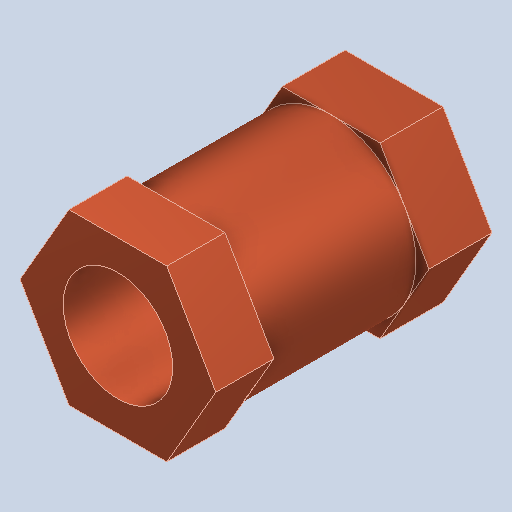
# Autodesk Inventor part: AcopleIntermedio
Saved by Autodesk Inventor 2023 (Build 270158000, 158)
## iProperties
Created: 2022-11-04
Part Number: AcopleIntermedio
Material: Copper
Document SubType Name: Modeling
Designer: Daniel Peña
Density: 8.94 g/cm^3
Appearance: Copper - Satin
Author: Daniel Peña
Autodesk Inventor part; units mm, degrees
ref_plane "YZ Plane" through (0, 0, 0) normal (1, 0, 0) x (0, 1, 0)
ref_plane "XZ Plane" through (0, 0, 0) normal (0, 1, 0) x (-1, 0, 0)
ref_plane "XY Plane" through (0, 0, 0) normal (0, 0, 1) x (1, 0, 0)
sketch "Sketch1" plane through (0, 0, 0) normal (0, 0, 1) x (1, 0, 0)
  line L0 (10.1036, 0) -> (5.0518, -8.75)
  line L1 (5.0518, -8.75) -> (-5.0518, -8.75)
  line L2 (-5.0518, -8.75) -> (-10.1036, 0)
  line L3 (-10.1036, 0) -> (-5.0518, 8.75)
  line L4 (-5.0518, 8.75) -> (5.0518, 8.75)
  line L5 (5.0518, 8.75) -> (10.1036, 0)
  circle A0 centre (0, 0) radius 5.5
  dimension "d0" = 17.5
  dimension "d1" = 11
  constraints: 12 end point, 2 coincident, 1 centre point, 13 other
  measures "d0" distance between parallel lines of L1 L4
  measures "d1" diameter of A0
extrude "Extrusion1" add sketch "Sketch1" along normal blind 6.5
sketch "Sketch2" plane through (0, 0, 6.5) normal (0, 0, 1) x (1, 0, 0)
  circle A0 centre (0, 0) radius 8.75
  circle A1 centre (0, 0) radius 5.65
  dimension "d4" = 17.5
  dimension "d5" = 11.3
  constraints: 2 centre point, 2 coincident
  measures "d4" diameter of A0
  measures "d5" diameter of A1
extrude "Extrusion2" add sketch "Sketch2" along normal blind 16
sketch "Sketch3" plane through (0, 0, 22.5) normal (0, 0, 1) x (1, 0, 0)
  circle A0 centre (0, 0) radius 5.65 projected
  line L0 (10.1036, 0) -> (5.0518, -8.75)
  line L1 (5.0518, -8.75) -> (-5.0518, -8.75)
  line L2 (-5.0518, -8.75) -> (-10.1036, 0)
  line L3 (-10.1036, 0) -> (-5.0518, 8.75)
  line L4 (-5.0518, 8.75) -> (5.0518, 8.75)
  line L5 (5.0518, 8.75) -> (10.1036, 0)
  dimension "d8" = 17.5
  constraints: 12 end point, 1 coincident, 13 other
  measures "d8" distance between parallel lines of L1 L4
extrude "Extrusion3" add sketch "Sketch3" along normal blind 6
body "Solid1"
